# Autodesk Inventor part: chicane
Saved by Autodesk Inventor 2021 (Build 250183000, 183)
## iProperties
Created: 2021-01-02
Part Number: chicane
Material: Generic
Document SubType Name: Modeling
Designer: Tomasz
Density: 1 g/cm^3
Appearance: Default
Mass: 2381.76 g
Surface Area: 15968.7 cm^2
Volume: 2381.76 cm^3
Author: Tomasz
Autodesk Inventor part; units mm, degrees
ref_plane "YZ Plane" through (0, 0, 0) normal (1, 0, 0) x (0, 1, 0)
ref_plane "XZ Plane" through (0, 0, 0) normal (0, 1, 0) x (-1, 0, 0)
ref_plane "XY Plane" through (0, 0, 0) normal (0, 0, 1) x (1, 0, 0)
sketch "Sketch1" plane through (0, 0, 0) normal (0, 1, 0) x (-1, 0, 0)
  line L0 (275, 0) -> (-275, 0)
  arc A0 (-275, 0) -> (-275, -360) centre (82.2114, -180) ccw
  arc A1 (-275, -720) -> (-275, -360) centre (-632.2114, -540) ccw
  arc A2 (-275, -720) -> (-275, -1080) centre (82.2114, -900) ccw
  arc A3 (-275, -1440) -> (-275, -1080) centre (-632.2114, -1260) ccw
  line L1 (-275, -1440) -> (275, -1440)
  line L2 (0, 0) -> (0, -1440) construction
  arc A4 (275, 0) -> (275, -360) centre (632.2114, -180) ccw
  arc A5 (275, -720) -> (275, -360) centre (-82.2114, -540) ccw
  arc A6 (275, -720) -> (275, -1080) centre (632.2114, -900) ccw
  arc A7 (275, -1440) -> (275, -1080) centre (-82.2114, -1260) ccw
  arc A8 (255, 0) -> (255, -360) centre (612.2114, -180) ccw
  arc A9 (255, -720) -> (255, -360) centre (-102.2114, -540) ccw
  arc A10 (255, -720) -> (255, -1080) centre (612.2114, -900) ccw
  arc A11 (255, -1440) -> (255, -1080) centre (-102.2114, -1260) ccw
  arc A12 (-255, 0) -> (-255, -360) centre (102.2114, -180) ccw
  arc A13 (-255, -720) -> (-255, -360) centre (-612.2114, -540) ccw
  arc A14 (-255, -720) -> (-255, -1080) centre (102.2114, -900) ccw
  arc A15 (-255, -1440) -> (-255, -1080) centre (-612.2114, -1260) ccw
  point P0 (255, 0)
  point P1 (-255, 0)
  dimension "d10" = 550
  dimension "d11" = 360
  dimension "d12" = 550
  dimension "d13" = 360
  dimension "d14" = 360
  dimension "d15" = 360
  dimension "d16" = 400
  dimension "d26" = 20
  dimension "d27" = 20
  constraints: 32 point on circle, 16 centre point, 16 equal radius, 15 vertical alignment, 12 horizontal alignment, 6 end point, 2 horizontal, 2 midpoint, 1 coincident
  measures "d10" distance of L0.start L0.end
  measures "d11" distance of A0.end L0.end
  measures "d12" distance of L1.start L1.end
  measures "d13" distance of A1.start A0.end
  measures "d14" distance of A2.end A1.start
  measures "d15" distance of L1.start A2.end
  measures "d16" radius of A0
  measures "d26" distance of L0.start A8.start
  measures "d27" distance of L0.end A12.start
extrude "Extrusion1" add sketch "Sketch1" along normal blind 3
extrude "Extrusion2" add sketch "Sketch1" along normal blind 3.1 contours A4 A5 A6 A7 L1 A11 A10 A9 A8 L0 | A12 A13 A14 A15 L1 A3 A2 A1 A0 L0
equation "\"d10\" = track_width"
equation "\"d12\" = d10"
equation "\"d13\" = d11"
equation "\"d14\" = d11"
equation "\"d15\" = d11"
equation "\"d26\" = d27"
equation "\"d27\" = curb_width"
equation "\"d22\" = track_height"
equation "\"d28\" = track_height + curb_height"
equation "\"track_width\" = 550"
equation "\"curb_width\" = 20"
equation "\"track_height\" = 3"
equation "\"curb_height\" = 0.1"
body "Solid1"
